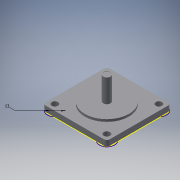
# Autodesk Inventor part: NEMA23
Saved by Autodesk Inventor 2016 (Build 200138000, 138)
## iProperties
Created: 2017-07-13
Part Number: NEMA23
Material: Generic
Document SubType Name: Modeling
Designer: ludwi
Density: 1 g/cm^3
Appearance: Default
Author: ludwi
Autodesk Inventor part; units mm, degrees
ref_plane "YZ Plane" through (0, 0, 0) normal (1, 0, 0) x (0, 1, 0)
ref_plane "XZ Plane" through (0, 0, 0) normal (0, 1, 0) x (-1, 0, 0)
ref_plane "XY Plane" through (0, 0, 0) normal (0, 0, 1) x (1, 0, 0)
sketch "Sketch1" plane through (0, 0, 0) normal (0, 0, 1) x (1, 0, 0)
  circle A0 centre (0, 0) radius 3.125
  dimension "d0" = 6.25
  constraints: 1 centre point, 1 coincident
  measures "d0" diameter of A0
extrude "Extrusion1" add sketch "Sketch1" along normal blind 20
sketch "Sketch2" plane through (0, 0, 0) normal (0, 0, -1) x (-1, 0, 0)
  circle A0 centre (0, 0) radius 19
  dimension "d3" = 38
  constraints: 1 centre point, 1 coincident
  measures "d3" diameter of A0
extrude "Extrusion2" add sketch "Sketch2" along normal blind 2
sketch "Sketch3" plane through (0, 0, -2) normal (0, 0, -1) x (-1, 0, 0)
  circle A0 centre (0, 0) radius 3.125 projected
  line L0 (27.75, 27.75) -> (-27.75, 27.75)
  line L1 (-27.75, 27.75) -> (-27.75, -27.75)
  line L2 (-27.75, -27.75) -> (27.75, -27.75)
  line L3 (27.75, -27.75) -> (27.75, 27.75)
  point P0 (27.75, 0)
  point P1 (0, 27.75)
  dimension "d6" = 55.5
  constraints: 8 end point, 2 midpoint, 2 parallel, 2 perpendicular, 1 horizontal, 1 horizontal alignment, 1 vertical alignment
  measures "d6" distance of L0.start L0.end
extrude "Extrusion3" add sketch "Sketch3" along normal blind 5
fillet "Fillet1" radius 2.5 4 edges at (27.75, 27.75, -4.5) (-27.75, 27.75, -4.5) (-27.75, -27.75, -4.5) (27.75, -27.75, -4.5)
sketch "Sketch4" plane through (0, 0, -2) normal (0, 0, 1) x (1, 0, 0)
  arc A0 (25.25, -27.75) -> (27.75, -25.25) centre (25.25, -25.25) ccw projected
  line L0 (27.75, 25.25) -> (27.75, -25.25) projected
  arc A1 (27.75, 25.25) -> (25.25, 27.75) centre (25.25, 25.25) ccw projected
  line L1 (-25.25, 27.75) -> (25.25, 27.75) projected
  arc A2 (-25.25, 27.75) -> (-27.75, 25.25) centre (-25.25, 25.25) ccw projected
  line L2 (-27.75, -25.25) -> (-27.75, 25.25) projected
  arc A3 (-27.75, -25.25) -> (-25.25, -27.75) centre (-25.25, -25.25) ccw projected
  line L3 (25.25, -27.75) -> (-25.25, -27.75) projected
  circle A4 centre (0, 0) radius 19 projected
  line L4 (-22.5, 22.5) -> (22.5, 22.5) construction
  line L5 (22.5, 22.5) -> (22.5, -22.5) construction
  line L6 (22.5, -22.5) -> (-22.5, -22.5) construction
  line L7 (-22.5, -22.5) -> (-22.5, 22.5) construction
  circle A5 centre (22.5, 22.5) radius 2.75
  circle A6 centre (-22.5, 22.5) radius 2.75
  circle A7 centre (-22.5, -22.5) radius 2.75
  circle A8 centre (22.5, -22.5) radius 2.75
  point P0 (-22.5, 0)
  point P1 (0, 22.5)
  dimension "d10" = 45
  dimension "d11" = 5.5
  constraints: 8 end point, 4 centre point, 4 coincident, 3 equal radius, 2 midpoint, 2 parallel, 2 perpendicular, 1 horizontal, 1 horizontal alignment, 1 vertical alignment
  measures "d10" distance of L4.start L4.end
  measures "d11" diameter of A5
extrude "Extrusion4" cut sketch "Sketch4" against normal through all contours A5 | A6 | A7 | A8
sketch "Sketch5" plane through (0, 0, -7) normal (0, 0, -1) x (-1, 0, 0)
  circle A0 centre (22.5, -22.5) radius 2.75 construction
  circle A1 centre (-22.5, 22.5) radius 2.75 construction
  circle A2 centre (22.5, 22.5) radius 2.75 construction
  circle A3 centre (-22.5, -22.5) radius 2.75 construction
  arc A4 (-27.75, -25.25) -> (-25.25, -27.75) centre (-25.25, -25.25) ccw construction
  line L0 (-25.25, -27.75) -> (25.25, -27.75) construction
  arc A5 (25.25, -27.75) -> (27.75, -25.25) centre (25.25, -25.25) ccw construction
  line L1 (27.75, -25.25) -> (27.75, 25.25) construction
  arc A6 (27.75, 25.25) -> (25.25, 27.75) centre (25.25, 25.25) ccw construction
  line L2 (25.25, 27.75) -> (-25.25, 27.75) construction
  arc A7 (-25.25, 27.75) -> (-27.75, 25.25) centre (-25.25, 25.25) ccw construction
  line L3 (-27.75, 25.25) -> (-27.75, -25.25) construction
  circle A8 centre (0, 0) radius 3.125 construction
  circle A9 centre (22.5, 22.5) radius 2.75 projected
  arc A10 (20.8606, 27.75) -> (27.75, 20.8606) centre (22.5, 22.5) ccw
  arc A11 (27.75, -20.8606) -> (20.8606, -27.75) centre (22.5, -22.5) ccw
  arc A12 (-20.8606, -27.75) -> (-27.75, -20.8606) centre (-22.5, -22.5) ccw
  arc A13 (-27.75, 20.8606) -> (-20.8606, 27.75) centre (-22.5, 22.5) ccw
  line L4 (27.75, 20.8606) -> (27.75, -20.8606)
  line L5 (20.8606, 27.75) -> (-20.8606, 27.75)
  line L6 (25.25, 27.75) -> (-25.25, 27.75) construction
  line L7 (-27.75, 20.8606) -> (-27.75, -20.8606)
  line L8 (-27.75, 25.25) -> (-27.75, -25.25) construction
  line L9 (-20.8606, -27.75) -> (20.8606, -27.75)
  dimension "d14" = 11
  constraints: 8 end point, 8 point on circle, 8 point on line, 4 centre point, 4 coincident, 3 collinear, 3 equal radius, 1 perpendicular
  measures "d14" diameter of A11
extrude "Extrusion5" add sketch "Sketch5" along normal blind 75 contours A10 L4 A11 L9 A12 L7 A13 L5
fillet "Fillet2" radius 2 8 edges at (20.8606, 27.75, -44.5) (27.75, 20.8606, -44.5) (-20.8606, 27.75, -44.5) (-27.75, 20.8606, -44.5) (20.8606, -27.75, -44.5) (27.75, -20.8606, -44.5) (-20.8606, -27.75, -44.5) (-27.75, -20.8606, -44.5)
body "Solid1"
